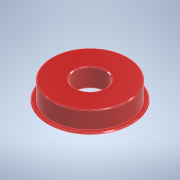
# Autodesk Inventor part: ベアリングフランジ付き
Saved by Autodesk Inventor 2021 (Build 250183000, 183)
## iProperties
Created: 2022-02-02
Part Number: ベアリングフランジ付き
Material: 一般
Document SubType Name: Modeling
Designer: hirohumi
Density: 1 g/cm^3
Appearance: 赤
Author: hirohumi
Autodesk Inventor part; units mm, degrees
ref_plane "YZ Plane" through (0, 0, 0) normal (1, 0, 0) x (0, 1, 0)
ref_plane "XZ Plane" through (0, 0, 0) normal (0, 1, 0) x (-1, 0, 0)
ref_plane "XY Plane" through (0, 0, 0) normal (0, 0, 1) x (1, 0, 0)
sketch "スケッチ1" plane through (0, 0, 0) normal (0, 0, 1) x (1, 0, 0)
  line L0 (4, 0) -> (4, 5)
  line L1 (4, 5) -> (10, 5)
  line L2 (10, 5) -> (10, 0.5)
  line L3 (10, 0.5) -> (11, 0.5)
  line L4 (11, 0.5) -> (11, 0)
  line L5 (11, 0) -> (4, 0)
  line L6 (0, 0) -> (0, 6.1022) construction
  dimension "d0" = 4
  dimension "d1" = 5
  dimension "d2" = 0.5
  dimension "d3" = 10
  dimension "d4" = 11
  constraints: 14 end point, 5 perpendicular, 2 vertical, 1 horizontal alignment
  measures "d0" distance from line of L0 L6.start
  measures "d1" distance between parallel lines of L5 L1
  measures "d2" distance between parallel lines of L5 L3
  measures "d3" distance from line of L6.start L2
  measures "d4" distance from line of L6.start L4
revolve "回転1" add sketch "スケッチ1" angle 360 about axis through (0, 0, 0) along (0, 1, 0)
chamfer "面取り1" distance 0.2 angle 45 5 edges at (-4, 5, 0) (-10, 5, 0) (-11, 0.5, 0) (-11, 0, 0) (-4, 0, 0)
